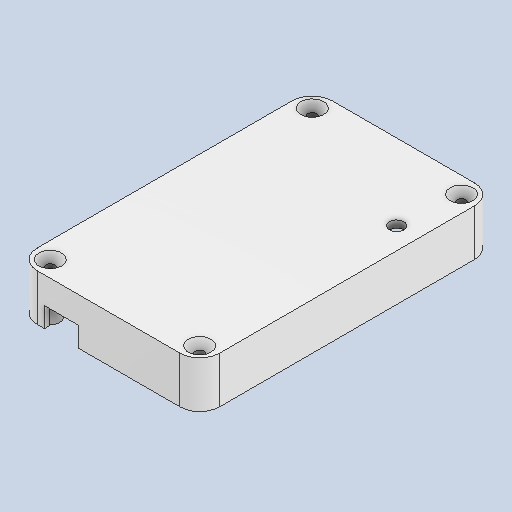
# Autodesk Inventor part: Крышка
Saved by Autodesk Inventor 2022 (Build 260153000, 153)
## iProperties
Created: 2022-01-08
Part Number: Крышка
Material: Пластик АБС
Document SubType Name: Modeling
Designer: user
Density: 1.06 g/cm^3
Appearance: Гладкий — белый
Mass: 13.0013 g
Surface Area: 148.998 cm^2
Volume: 12.2654 cm^3
Author: user
Autodesk Inventor part; units mm, degrees
ref_plane "YZ Plane" through (0, 0, 0) normal (1, 0, 0) x (0, 1, 0)
ref_plane "XZ Plane" through (0, 0, 0) normal (0, 1, 0) x (-1, 0, 0)
ref_plane "XY Plane" through (0, 0, 0) normal (0, 0, 1) x (1, 0, 0)
sketch "Эскиз1" plane through (0, 0, 0) normal (0, 1, 0) x (-1, 0, 0)
  circle A0 centre (0, 0) radius 2.5
  circle A1 centre (0, -72.634) radius 2.5
  circle A2 centre (-41.385, 0) radius 2.5
  circle A3 centre (-41.385, -72.634) radius 2.5
  dimension "d1" = 5
  dimension "d3" = 5
  dimension "d5" = 5
  dimension "d7" = 5
  constraints: 4 centre point
  measures "d1" diameter of A0
  measures "d3" diameter of A1
  measures "d5" diameter of A2
  measures "d7" diameter of A3
extrude "Выдавливание1" add sketch "Эскиз1" along normal blind 12
sketch "Эскиз2" plane through (41.385, 12, 0) normal (0, 1, 0) x (1, 0, 0)
  arc A0 (-44.6516, 0.8672) -> (-40.4502, -3.3343) centre (-40.4502, 0.8672) ccw
  arc A1 (-40.4599, 75.8769) -> (-44.6537, 71.6872) centre (-40.462, 71.6851) ccw
  arc A2 (3.3348, 71.7001) -> (-0.8419, 75.8769) centre (-0.8419, 71.7001) ccw
  arc A3 (-0.8516, -3.3343) -> (3.3348, 0.8657) centre (-0.8652, 0.8657) ccw
  line L0 (-40.4502, -3.3343) -> (-0.8516, -3.3343)
  line L1 (3.3348, 0.8657) -> (3.3348, 71.7001)
  line L2 (-0.8419, 75.8769) -> (-40.4599, 75.8769)
  arc A4 (-45.9516, 0.8672) -> (-40.4502, -4.6343) centre (-40.4502, 0.8672) ccw
  arc A5 (4.6083, 71.6927) -> (-0.8706, 77.1655) centre (-0.8679, 71.6894) ccw
  arc A6 (-0.8516, -4.6343) -> (4.6517, 0.8657) centre (-0.8513, 0.8687) ccw
  line L3 (-45.9516, 0.8672) -> (-45.9516, 71.5214)
  line L4 (-40.4886, 77.1457) -> (-0.8706, 77.1655)
  line L5 (4.6083, 71.6927) -> (4.6517, 0.8739)
  line L6 (-0.8516, -4.6343) -> (-40.4502, -4.6343)
  line L7 (-44.6516, 0.8672) -> (-44.6537, 71.6872)
  circle A7 centre (0, 72.634) radius 1.5
  circle A8 centre (0, 72.634) radius 1.5 projected
  line L8 (4.6517, 0.8739) -> (4.6517, 0.8657)
  line L9 (-40.4886, 77.1457) -> (-24.1126, 77.1457) construction
  arc A9 (-40.4886, 77.1457) -> (-45.9516, 71.5214) centre (-40.3249, 71.5214) ccw
  point P0 (-41.385, 0)
  constraints: 20 end point, 16 point on circle, 9 centre point, 3 horizontal, 2 tangent, 1 perpendicular, 1 vertical
extrude "Выдавливание2" add sketch "Эскиз2" along normal blind 2 contours L7 A1 L2 A2 L1 A3 L0 A0 | L3 A9 L4 A5 L5 L8 A6 L6 A4 | A7
sketch "Эскиз4" plane through (41.385, 12, 0) normal (0, -1, 0) x (1, 0, 0)
  arc A0 (-44.6516, -71.7668) -> (-40.4502, -75.9683) centre (-40.4502, -71.7668) ccw
  arc A1 (-40.4599, 3.2429) -> (-44.6537, -0.9468) centre (-40.462, -0.9489) ccw
  arc A2 (3.3348, -0.9339) -> (-0.8419, 3.2429) centre (-0.8419, -0.9339) ccw
  arc A3 (-0.8516, -75.9683) -> (3.3348, -71.7683) centre (-0.8652, -71.7683) ccw
  line L0 (-40.4502, -75.9683) -> (-0.8516, -75.9683)
  line L1 (3.3348, -71.7683) -> (3.3348, -0.9339)
  line L2 (-0.8419, 3.2429) -> (-40.4599, 3.2429)
  line L3 (-44.6516, -71.7668) -> (-44.6537, -0.9468)
  arc A4 (4.6517, -0.8739) -> (-0.8516, 4.6343) centre (-0.8513, -0.8687) ccw projected
  line L4 (-0.8706, -77.1655) -> (-40.4886, -77.1457) projected
  line L5 (-40.4886, -77.1457) -> (-0.8706, -77.1655)
  arc A5 (-45.9516, -71.5214) -> (-40.4886, -77.1457) centre (-40.3249, -71.5214) ccw projected
  line L6 (-45.9516, -71.5214) -> (-45.9516, -0.8739)
  line L7 (-40.4502, 4.6343) -> (-0.8516, 4.6343) projected
  line L8 (-40.4502, 4.6343) -> (-0.8516, 4.6343)
  arc A6 (4.6517, -0.8739) -> (-0.8516, 4.6343) centre (-0.8513, -0.8687) ccw
  arc A7 (-0.8706, -77.1655) -> (4.6083, -71.6927) centre (-0.8679, -71.6894) ccw projected
  line L9 (4.6083, -71.6927) -> (4.6517, -0.8739)
  arc A8 (-0.8706, -77.1655) -> (4.6083, -71.6927) centre (-0.8679, -71.6894) ccw projected
  line L10 (4.6517, -0.8739) -> (4.6083, -71.6927) projected
  arc A9 (-0.8706, -77.1655) -> (4.6083, -71.6927) centre (-0.8679, -71.6894) ccw
  arc A10 (-45.9516, -71.5214) -> (-40.4886, -77.1457) centre (-40.3249, -71.5214) ccw projected
  arc A11 (-40.4502, 4.6343) -> (-45.9516, -0.8672) centre (-40.4502, -0.8672) ccw projected
  arc A12 (-40.4502, 4.6343) -> (-45.9516, -0.8672) centre (-40.4502, -0.8672) ccw
  arc A13 (-45.9516, -71.5214) -> (-40.4886, -77.1457) centre (-40.3249, -71.5214) ccw
  arc A14 (-40.4502, 4.6343) -> (-45.9516, -0.8672) centre (-40.4502, -0.8672) ccw projected
  line L11 (-45.9516, -0.8739) -> (-45.9516, -0.8672)
  point P0 (-41.385, 0)
  constraints: 18 end point, 16 point on circle, 8 centre point, 7 tangent, 2 concentric, 2 horizontal, 2 vertical, 1 coincident, 1 collinear, 1 perpendicular
extrude "Выдавливание4" add sketch "Эскиз4" along normal blind 10.911
sketch "Эскиз5" plane through (-4.5666, 14, -71.5214) normal (-1, 0, 0) x (0, 0, 1)
  line L0 (11.3757, -6.5285) -> (21.3757, -6.5285)
  line L1 (21.3757, -6.5285) -> (21.3757, -11.8804)
  line L2 (21.3757, -11.8804) -> (11.3757, -11.8804)
  line L3 (11.3757, -11.8804) -> (11.3757, -6.5285)
  line L4 (-5.6243, -12.911) -> (-5.6243, 0) projected
  line L5 (26.3757, -6.4555) -> (40.3757, -6.4555)
  line L6 (40.3757, -6.4555) -> (40.3757, -11.8804)
  line L7 (40.3757, -11.8804) -> (26.3757, -11.8804)
  line L8 (26.3757, -11.8804) -> (26.3757, -6.4555)
  point P0 (71.5214, -14)
  dimension "d19" = 17
  dimension "d20" = 27
  dimension "d23" = 32
  dimension "d24" = 46
  constraints: 16 end point, 4 parallel, 2 horizontal, 2 perpendicular
  measures "d19" distance between parallel lines of L4 L3
  measures "d20" distance between parallel lines of L1 L4
  measures "d23" distance between parallel lines of L8 L4
  measures "d24" distance between parallel lines of L6 L4
extrude "Выдавливание5" cut sketch "Эскиз5" against normal blind 10
sketch "Эскиз6" plane through (0.9348, 14, 4.6343) normal (0, 0, 1) x (1, 0, 0)
  line L0 (1.9985, -7.3816) -> (11.4985, -7.3816)
  line L1 (11.4985, -7.3816) -> (11.4985, -13.551)
  line L2 (11.4985, -13.551) -> (1.9985, -13.551)
  line L3 (1.9985, -13.551) -> (1.9985, -7.3816)
  line L4 (-5.5015, -12.911) -> (-5.5015, 0) projected
  point P0 (-0.9348, -14)
  dimension "d25" = 7.5
  dimension "d26" = 17
  constraints: 8 end point, 2 parallel, 1 horizontal, 1 perpendicular
  measures "d25" distance between parallel lines of L3 L4
  measures "d26" distance between parallel lines of L4 L1
extrude "Выдавливание6" cut sketch "Эскиз6" against normal blind 10
sketch "Эскиз7" plane through (41.385, 14, 0) normal (0, 1, 0) x (1, 0, 0)
  line L0 (-0.8706, 77.1655) -> (-40.4886, 77.1457) projected
  line L1 (4.6083, 71.6927) -> (4.6517, 0.8739) projected
  circle A0 centre (-1.3917, 56.0655) radius 2
  point P0 (-41.385, 0)
  dimension "d31" = 4
  constraints: 1 centre point
  measures "d31" diameter of A0
extrude "Выдавливание7" cut sketch "Эскиз7" against normal blind 10
sketch "Эскиз8" plane through (41.385, 14, 0) normal (0, 1, 0) x (1, 0, 0)
  point P0 (-41.3846, 72.6332)
hole "Отверстие1" at (0.0004, 14, -72.6332) direction (0, -1, 0) diameter 2.459 depth 21.1198 tip angle 120 countersink diameter 6.3 countersink angle 90 thread size "M3x0.5" class "6H" standard "ISO Metric profile"
sketch "Эскиз9" plane through (41.385, 14, 0) normal (0, 1, 0) x (1, 0, 0)
  point P0 (0.0407, 72.654)
hole "Отверстие2" at (41.4257, 14, -72.654) direction (0, -1, 0) diameter 2.459 depth 21.1847 tip angle 120 countersink diameter 6.3 countersink angle 90 thread size "M3x0.5" class "6H" standard "ISO Metric profile"
sketch "Эскиз10" plane through (41.385, 14, 0) normal (0, 1, 0) x (1, 0, 0)
  point P0 (0.0853, -0.1223)
hole "Отверстие3" at (41.4703, 14, 0.1223) direction (0, -1, 0) diameter 2.459 depth 21.5662 tip angle 120 countersink diameter 6.3 countersink angle 90 thread size "M3x0.5" class "6H" standard "ISO Metric profile"
sketch "Эскиз11" plane through (41.385, 14, 0) normal (0, 1, 0) x (1, 0, 0)
  point P0 (-41.3846, -0.1223)
hole "Отверстие4" at (0.0004, 14, 0.1223) direction (0, -1, 0) diameter 2.459 depth 21.6826 tip angle 120 countersink diameter 6.3 countersink angle 90 thread size "M3x0.5" class "6H" standard "ISO Metric profile"
